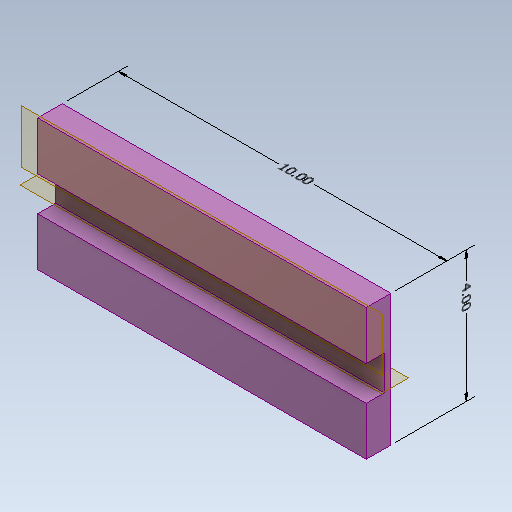
# Autodesk Inventor part: pistonHousing-8-in
Saved by Autodesk Inventor 2020.2 (Build 242310000, 310)
## iProperties
Created: 2020-01-13
Part Number: pistonHousing-8-in
Material: PET Plastic
Document SubType Name: Modeling
Designer: robst
Density: 1.541 g/cm^3
Appearance: Smooth - Purple
Author: robst
Autodesk Inventor part; units mm, degrees
ref_plane "YZ Plane" through (0, 0, 0) normal (1, 0, 0) x (0, 1, 0)
ref_plane "XY Plane" through (0, 0, 0) normal (0, 0, 1) x (1, 0, 0)
sketch "Sketch1" plane through (0, 0, 0) normal (0, 0, 1) x (1, 0, 0)
  line L0 (-127, -50.8) -> (127, -50.8)
  line L1 (127, -50.8) -> (127, 50.8)
  line L2 (127, 50.8) -> (-127, 50.8)
  line L3 (-127, 50.8) -> (-127, -50.8)
  line L4 (-127, -50.8) -> (127, 50.8) construction
  line L5 (127, -50.8) -> (-127, 50.8) construction
  point P0 (0, 0)
  dimension "d0" = 254
  dimension "d1" = 101.6
  constraints: 12 end point, 2 midpoint, 2 parallel, 1 horizontal, 1 perpendicular
  measures "d0" distance of L2.end L1.end
  measures "d1" distance of L1.end L0.end
extrude "Extrusion1" add sketch "Sketch1" along normal mid plane 19.05
sketch "Sketch10" plane through (0, 0, 9.525) normal (0, 0, 1) x (1, 0, 0)
  line L0 (-127, -13.335) -> (127, -13.335)
  line L1 (127, -13.335) -> (127, 13.335)
  line L2 (127, 13.335) -> (-127, 13.335)
  line L3 (-127, 13.335) -> (-127, -13.335)
  line L4 (-127, -13.335) -> (127, 13.335) construction
  line L5 (127, -13.335) -> (-127, 13.335) construction
  point P0 (0, 0)
  dimension "d71" = 26.67
  constraints: 12 end point, 2 midpoint, 2 parallel, 1 perpendicular
  measures "d71" distance of L1.end L0.end
extrude "Extrusion7" cut sketch "Sketch10" against normal blind 13.97
ref_plane "Work Plane3" through (0, 0, 0) normal (0, 0, 1) x (1, 0, 0)
ref_plane "Work Plane4" through (0, 0, 9.525) normal (0, 0, 1) x (1, 0, 0)
sketch "Sketch3" plane through (0, 0, 9.525) normal (0, 0, 1) x (1, 0, 0)
  line L0 (-76.2, -12.7) -> (76.2, -12.7)
  line L1 (76.2, -12.7) -> (76.2, 12.7)
  line L2 (76.2, 12.7) -> (-76.2, 12.7)
  line L3 (-76.2, 12.7) -> (-76.2, -12.7)
  line L4 (-76.2, -12.7) -> (76.2, 12.7) construction
  line L5 (76.2, -12.7) -> (-76.2, 12.7) construction
  point P0 (0, 0)
  dimension "d7" = 25.4
  dimension "d19" = 152.4
  constraints: 12 end point, 2 midpoint, 2 parallel, 1 horizontal, 1 perpendicular
  measures "d7" distance of L1.end L0.end
  measures "d19" distance of L1.end L2.end
sketch "Sketch8" plane through (0, 0, 9.525) normal (0, 0, 1) x (1, 0, 0)
  line L0 (-76.2, -12.7) -> (-76.2, 12.7) projected
  line L1 (-76.2, 0) -> (38.1, 0)
  line L2 (38.1, 0) -> (38.1, 38.1)
  line L3 (38.1, 38.1) -> (-76.2, 38.1)
  line L4 (-76.2, 38.1) -> (-76.2, 0)
  line L5 (38.1, 0) -> (38.1, -38.1)
  line L6 (38.1, -38.1) -> (-76.2, -38.1)
  line L7 (-76.2, -38.1) -> (-76.2, 0)
  point P0 (0, 0)
  dimension "d51" = 114.3
  dimension "d52" = 38.1
  constraints: 14 end point, 2 parallel, 2 symmetric about line, 1 horizontal, 1 midpoint, 1 perpendicular
  measures "d51" distance of L3.end L2.end
  measures "d52" distance of L2.end L1.end
sketch "Sketch9" plane through (0, 0, 9.525) normal (0, 0, 1) x (1, 0, 0)
  line L0 (-127, 50.8) -> (-127, -50.8) construction
  line L1 (-127, -57.15) -> (127, -57.15) construction
  line L2 (127, 50.8) -> (127, -50.8) construction
  line L3 (-127, -57.15) -> (-127, -44.4609) construction
  point P0 (0, 0)
  point P1 (-76.2, 38.1)
  point P2 (-101.6, -57.15)
  point P3 (-76.2, -57.15)
  point P4 (-50.8, -57.15)
  point P5 (-25.4, -57.15)
  point P6 (0, -57.15)
  point P7 (-101.6, -146.05)
  point P8 (-76.2, -146.05)
  point P9 (-50.8, -146.05)
  point P10 (-25.4, -146.05)
  point P11 (0, -146.05)
  point P12 (-101.6, -234.95)
  point P13 (-76.2, -234.95)
  point P14 (-50.8, -234.95)
  point P15 (-25.4, -234.95)
  point P16 (0, -234.95)
  point P17 (-101.6, -323.85)
  point P18 (-76.2, -323.85)
  point P19 (-50.8, -323.85)
  point P20 (-25.4, -323.85)
  point P21 (0, -323.85)
  dimension "d55" = 25.4
  dimension "d58" = 25.4
  dimension "d61" = 88.9
  constraints: 4 end point, 2 horizontal, 2 point on line, 2 vertical, 21 other
  measures "d58" distance of point (-101.6, -57.15) point (-76.2, -57.15)
  measures "d61" distance of point (-101.6, -57.15) point (-101.6, -146.05)
body "Solid1"
